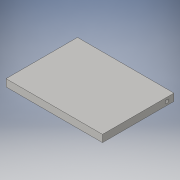
# Autodesk Inventor part: STEP
Saved by Autodesk Inventor 2016 (Build 200138000, 138)
## iProperties
Created: 2019-01-25
Part Number: STEP
Material: Generic
Document SubType Name: Modeling
Designer: Matthew Reese
Density: 1 g/cm^3
Appearance: Default
Author: Matthew Reese
Autodesk Inventor part; units mm, degrees
ref_plane "YZ Plane" through (0, 0, 0) normal (1, 0, 0) x (0, 1, 0)
ref_plane "XZ Plane" through (0, 0, 0) normal (0, 1, 0) x (-1, 0, 0)
ref_plane "XY Plane" through (0, 0, 0) normal (0, 0, 1) x (1, 0, 0)
sketch "Sketch1" plane through (0, 0, 0) normal (0, 1, 0) x (-1, 0, 0)
  line L0 (171.45, 127) -> (-171.45, 127)
  line L1 (-171.45, 127) -> (-171.45, -127)
  line L2 (-171.45, -127) -> (171.45, -127)
  line L3 (171.45, -127) -> (171.45, 127)
  line L4 (171.45, 127) -> (-171.45, -127) construction
  line L5 (-171.45, 127) -> (171.45, -127) construction
  point P0 (0, 0)
  dimension "d0" = 342.9
  dimension "d1" = 254
  constraints: 12 end point, 2 midpoint, 2 parallel, 1 horizontal, 1 perpendicular
  measures "d0" distance of L2.end L1.end
  measures "d1" distance of L1.end L0.end
extrude "Extrusion1" add sketch "Sketch1" along normal blind 25.4
sketch "Sketch6" plane through (171.45, 0, 127) normal (1, 0, 0) x (0, 0, -1)
  line L0 (0, 25.4) -> (254, 25.4) projected
  line L1 (254, 0) -> (254, 25.4) projected
  point P0 (127, 0)
  point P1 (228.6, 12.7)
  dimension "d18" = 25.4
  dimension "d19" = 12.7
  measures "d18" distance from line of point (228.6, 12.7) L1
  measures "d19" distance from line of point (228.6, 12.7) L0
hole "Hole2" at (171.45, 12.7, -101.6) direction (-1, 0, 0) diameter 12.7 depth 12.7
sketch "Sketch8" plane through (-171.45, 0, -127) normal (-1, 0, 0) x (0, 0, 1)
  circle A0 centre (25.4, 12.7) radius 6.35 projected
  point P0 (127, 0)
  constraints: 1 coincident
hole "Hole3" at (-171.45, 12.7, -101.6) direction (1, 0, 0) diameter 12.7 depth 12.7
body "Solid1"
